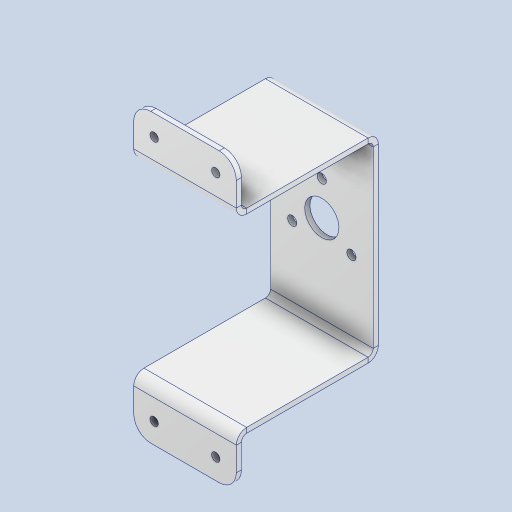
# Autodesk Inventor part: hand_box2
Saved by Autodesk Inventor 2023 (Build 270158000, 158)
## iProperties
Created: 2024-12-05
Part Number: hand_box2
Material: アルミニウム 6061
Document SubType Name: Sheet Metal
Designer: kiyo
Density: 2.7 g/cm^3
Sheet Metal Rule: Default_mm
Appearance: アルミニウム - フラット
Author: kiyo
Autodesk Inventor part; units mm, degrees
ref_plane "YZ Plane" through (0, 0, 0) normal (1, 0, 0) x (0, 1, 0)
ref_plane "XZ Plane" through (0, 0, 0) normal (0, 1, 0) x (-1, 0, 0)
ref_plane "XY Plane" through (0, 0, 0) normal (0, 0, 1) x (1, 0, 0)
sketch "スケッチ1" plane through (0, 0, 0) normal (1, 0, 0) x (0, 1, 0)
  line L0 (-15, -27) -> (-15, 27)
  line L1 (-15, 27) -> (15, 27)
  line L2 (15, 27) -> (15, -27)
  line L3 (15, -27) -> (-15, -27)
  line L4 (-15, -27) -> (15, 27) construction
  line L5 (-15, 27) -> (15, -27) construction
  point P0 (0, 0)
  dimension "d0" = 30
  dimension "d1" = 54
  measures "d0" distance of L0.end L1.end
  measures "d1" distance of L0.start L0.end
extrude "プレート1" add sketch "スケッチ1" along normal blind 1.5
sketch "スケッチ2" plane through (1.5, -15, 27) normal (0, 0, 1) x (1, 0, 0)
  line L0 (0, 30) -> (0, 0)
  line L1 (0, 0) -> (38.5, 0)
  line L2 (38.5, 0) -> (38.5, 30)
  line L3 (38.5, 30) -> (0, 30)
  constraints: 6 end point, 1 horizontal, 1 perpendicular, 1 vertical
edge flange "フランジ1" height 40 angle 90 thickness 1.5 bend radius 1.5 thickness toward (0, 0, 1) relief straight relief width 1.5 relief depth 0.75 corner gap 1.5 corner form 0 edges at (1.5, 0, 27) (1.5, 0, -27) wall of the first edge with corners at (1.5, 15, 27) (1.5, -15, 27) (40, -15, 27) (40, 15, 27)
bend "曲げ1"
corner "コーナー1"
sketch "スケッチ3" plane through (40, 15, 28.5) normal (1, 0, 0) x (0, 1, 0)
  line L0 (-30, 0) -> (0, 0)
  line L1 (0, 0) -> (0, 13.5)
  line L2 (0, 13.5) -> (-30, 13.5)
  line L3 (-30, 13.5) -> (-30, 0)
  constraints: 6 end point, 1 horizontal, 1 perpendicular, 1 vertical
edge flange "フランジ2" height 15 angle 90 thickness 1.5 bend radius 1.5 thickness toward (1, 0, 0) relief straight relief width 1.5 relief depth 0.75 corner gap 1.5 corner form 0 edges at (40, 0, 28.5) (40, 0, -28.5) wall of the first edge with corners at (40, -15, 28.5) (40, 15, 28.5) (40, 15, 42) (40, -15, 42)
bend "曲げ2"
corner "コーナー2"
sketch "スケッチ4" plane through (0, 0, 0) normal (-1, 0, 0) x (0, 0, 1)
  circle A0 centre (0, 0) radius 5
  circle A1 centre (10, 0) radius 1.35
  circle A2 centre (-5, 8.6603) radius 1.35
  circle A3 centre (-5, -8.6603) radius 1.35
  dimension "d23" = 10
  dimension "d24" = 2.7
  dimension "d25" = 0
  dimension "d26" = 10
  dimension "d29" = 360
  constraints: 4 centre point, 1 coincident, 7 other
  measures "d23" diameter of A0
  measures "d24" diameter of A1
  measures "d25" vertical distance of point (0, 0) A1.centre
  measures "d26" distance of A0.centre A1.centre
extrude "押し出し1" cut sketch "スケッチ4" against normal blind 2
sketch "スケッチ6" plane through (40, -15, 42) normal (-1, 0, 0) x (0, 0, 1)
  circle A0 centre (-6, 24) radius 2
  line L0 (-12, 30) -> (0, 30) projected
  line L1 (0, 0) -> (0, 30) projected
  circle A1 centre (-6, 6) radius 2
  circle A2 centre (-78, 24) radius 2
  circle A3 centre (-78, 6) radius 2
  point P0 (-42, 15)
  dimension "d41" = 4
  dimension "d42" = 4
  dimension "d43" = 4
  dimension "d46" = 18
  dimension "d49" = 72
  constraints: 4 centre point, 1 horizontal, 1 vertical, 6 other
  measures "d41" diameter of A0
  measures "d42" distance edge to line of A0 L0
  measures "d43" distance edge to line of A0 L1
  measures "d46" distance of A0.centre A1.centre
  measures "d49" distance of A0.centre A2.centre
extrude "押し出し3" add sketch "スケッチ6" along normal blind 1.5
sketch "スケッチ7" plane through (38.5, 9, 36) normal (-1, 0, 0) x (0, 0, 1)
  circle A0 centre (0, 0) radius 2 projected
  circle A1 centre (0, -18) radius 2 projected
  circle A2 centre (-72, -18) radius 2 projected
  circle A3 centre (-72, 0) radius 2 projected
  circle A4 centre (0, 0) radius 2 projected
  circle A5 centre (0, -18) radius 2 projected
  circle A6 centre (-72, -18) radius 2 projected
  point P0 (-36, -9)
  constraints: 4 coincident
hole "穴1" at (38.5, 9, 36) at (38.5, -9, 36) at (38.5, 9, -36) at (38.5, -9, -36) direction (1, 0, 0) diameter 2.459 depth 3 tip angle 118 thread size "M3x0.5" designation "M3" class "6H" standard "GB Metric profile"
fillet "フィレット1" radius 5 4 edges at (40.75, 15, 42) (40.75, -15, 42) (40.75, 15, -42) (40.75, -15, -42)
equation "\"d59\" = Thickness"
equation "\"BendRadius\" = Thickness"
equation "\"BendReliefWidth\" = Thickness"
equation "\"BendReliefDepth\" = 0.5 * Thickness"
equation "\"CornerReliefSize\" = 4 * Thickness"
equation "\"MinimumRemnant\" = 2 * Thickness"
equation "\"TransitionRadius\" = BendRadius"
equation "\"JacobiRadiusSize\" = BendRadius"
equation "\"GapSize\" = Thickness"
